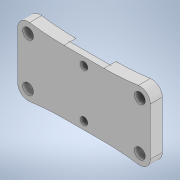
# Autodesk Inventor part: AS5600HolderV2
Saved by Autodesk Inventor 2022 (Build 260153070, 153G)
## iProperties
Created: 2022-01-12
Part Number: AS5600HolderV2
Material: Generic
Document SubType Name: Modeling
Designer: a laptop
Density: 1 g/cm^3
Appearance: Default
Author: a laptop
Autodesk Inventor part; units mm, degrees
ref_plane "YZ Plane" through (0, 0, 0) normal (1, 0, 0) x (0, 1, 0)
ref_plane "XZ Plane" through (0, 0, 0) normal (0, 1, 0) x (-1, 0, 0)
ref_plane "XY Plane" through (0, 0, 0) normal (0, 0, 1) x (1, 0, 0)
sketch "Sketch1" plane through (0, 0, 0) normal (0, 0, 1) x (1, 0, 0)
  circle A0 centre (0, 6) radius 0.95
  circle A1 centre (0, -6) radius 0.95
  line L0 (0, 6) -> (0, -6) construction
  line L1 (5, 7.95) -> (-5, 7.95)
  line L2 (-5, 7.95) -> (-5, -7.95) construction
  line L3 (-5, -7.95) -> (5, -7.95)
  line L4 (5, -7.95) -> (5, 7.95) construction
  circle A2 centre (14, 6) radius 1.35
  circle A3 centre (14, -6) radius 1.35
  circle A4 centre (-14, 6) radius 1.35
  circle A5 centre (-14, -6) radius 1.35
  circle A6 centre (-14, 6) radius 2.6
  arc A7 (-13.6264, 8.573) -> (-5, 7.95) centre (-5, 67.9827) ccw
  circle A8 centre (-14, -6) radius 2.6
  circle A9 centre (14, 6) radius 2.6
  circle A10 centre (14, -6) radius 2.6
  line L5 (-16.6, 6) -> (-16.6, -6)
  arc A11 (5, 7.95) -> (13.6264, 8.573) centre (5, 67.9827) ccw
  line L6 (16.6, 6) -> (16.6, -6)
  arc A12 (-5, -7.95) -> (-13.6264, -8.573) centre (-5, -67.9827) ccw
  arc A13 (13.6264, -8.573) -> (5, -7.95) centre (5, -67.9827) ccw
  line L7 (10, 8.1586) -> (10, -8.1586)
  line L8 (-10, -8.1586) -> (-10, 8.1586)
  arc A14 (5, -7.95) -> (10, -2.95) centre (5, -2.95) ccw
  arc A15 (10, 2.95) -> (5, 7.95) centre (5, 2.95) ccw
  arc A16 (-10, -2.95) -> (-5, -7.95) centre (-5, -2.95) ccw
  arc A17 (-5, 7.95) -> (-10, 2.95) centre (-5, 2.95) ccw
  point P0 (0, 0)
  point P1 (0, 0)
  dimension "d0" = 1.9
  dimension "d1" = 1.9
  dimension "d2" = 12
  dimension "d3" = 1.95
  dimension "d4" = 1.95
  dimension "d5" = 5
  dimension "d6" = 5
  dimension "d7" = 2.7
  dimension "d8" = 14
  dimension "d9" = 14
  dimension "d10" = 1.25
  dimension "d11" = 10
  dimension "d12" = 10
  constraints: 28 point on circle, 19 tangent, 18 centre point, 18 end point, 6 equal radius, 4 horizontal alignment, 4 point on line, 3 concentric, 3 vertical, 2 coincident, 2 parallel, 2 vertical alignment, 1 horizontal, 1 midpoint, 1 perpendicular
  measures "d0" diameter of A0
  measures "d1" diameter of A1
  measures "d2" distance of L0.start L0.end
  measures "d3" distance from line of L0.start L1
  measures "d4" distance from line of L3 L0.end
  measures "d5" distance between parallel lines of L4 L0
  measures "d6" distance between parallel lines of L2 L0
  measures "d7" diameter of A2
  measures "d8" distance of A2.centre L0.start
  measures "d9" distance from line of A4.centre L0
  measures "d10" radial gap between concentric circles of A4 A6
  measures "d11" distance between parallel lines of L0 L7
  measures "d12" distance from line of point (0, 0) L8
extrude "Extrusion1" add sketch "Sketch1" along normal blind 1.5
extrude "Extrusion2" add sketch "Sketch1" against normal blind 1.5 contours A11 L7 A15 | A17 L8 A7 | A11 A9 L6 A10 A13 L7 | L8 A12 A8 L5 A6 A7 | A9 | L7 A13 A14 | A6 | A16 A12 L8 | A10 | A8
body "Solid1"
